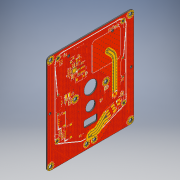
# Autodesk Inventor part: +XPanel_PCB
Saved by Autodesk Inventor 2018 (Build 220112000, 112)
## iProperties
Created: 2018-10-25
Part Number: +XPanel_PCB
Material: Epoxy Resin
Document SubType Name: Modeling
Designer: Bradley
Density: 1.14 g/cm^3
Appearance: Smooth - Dark Gray
Author: Bradley
Autodesk Inventor part; units mm, degrees
ref_plane "YZ Plane" through (0, 0, 0) normal (1, 0, 0) x (0, 1, 0)
ref_plane "XZ Plane" through (0, 0, 0) normal (0, 1, 0) x (-1, 0, 0)
ref_plane "XY Plane" through (0, 0, 0) normal (0, 0, 1) x (1, 0, 0)
sketch "Sketch1" plane through (0, 0, 0) normal (1, 0, 0) x (0, 1, 0)
  line L0 (36.5, -42) -> (-36.5, -42) construction
  line L1 (-36.5, -42) -> (-36.5, 42) construction
  line L2 (-36.5, 42) -> (36.5, 42) construction
  line L3 (36.5, 42) -> (36.5, -42) construction
  line L4 (36.5, -42) -> (-36.5, 42) construction
  line L5 (-36.5, -42) -> (36.5, 42) construction
  line L6 (-14, 0) -> (14, 0) construction
  line L7 (-39.5, -42) -> (-39.5, 42)
  arc A0 (-36.5, 45) -> (-39.5, 42) centre (-36.5, 42) ccw
  line L8 (-36.5, 45) -> (36.5, 45)
  arc A1 (39.5, 42) -> (36.5, 45) centre (36.5, 42) ccw
  line L9 (39.5, 42) -> (39.5, -42)
  arc A2 (36.5, -45) -> (39.5, -42) centre (36.5, -42) ccw
  line L10 (36.5, -45) -> (-36.5, -45)
  arc A3 (-39.5, -42) -> (-36.5, -45) centre (-36.5, -42) ccw
  point P0 (0, 0)
  point P1 (0, 0)
  dimension "d2" = 28
  dimension "d3" = 79
  dimension "d117" = 3
  dimension "d118" = 90
  dimension "d119" = 84
  dimension "d120" = 73
  constraints: 22 end point, 8 point on circle, 6 tangent, 4 centre point, 4 coincident, 4 midpoint, 4 parallel, 2 horizontal, 2 perpendicular, 1 equal radius, 1 vertical
  measures "d2" distance of L6.start L6.end
  measures "d3" distance between parallel lines of L9 L7
  measures "d117" radius of A0
  measures "d118" distance between parallel lines of L10 L8
  measures "d119" distance of L0.end L1.end
  measures "d120" distance of L1.end L2.end
extrude "Extrusion1" add sketch "Sketch1" along normal mid plane 1
sketch "Sketch3" plane through (0.5, 0, 0) normal (1, 0, 0) x (0, 0, -1)
  circle A0 centre (-2.5, 0) radius 6
  circle A1 centre (12.35, 0) radius 4.5
  line L0 (26, -6) -> (22, -6)
  line L1 (21, -5) -> (21, 5)
  line L2 (22, 6) -> (26, 6)
  line L3 (27, 5) -> (27, -5)
  line L4 (27, -6) -> (21, 6) construction
  line L5 (21, -6) -> (27, 6) construction
  arc A2 (21, -5) -> (22, -6) centre (22, -5) ccw
  arc A3 (26, -6) -> (27, -5) centre (26, -5) ccw
  arc A4 (27, 5) -> (26, 6) centre (26, 5) ccw
  arc A5 (22, 6) -> (21, 5) centre (22, 5) ccw
  point P0 (0, 0)
  point P1 (24, 0)
  point P2 (24, 0)
  dimension "d15" = 2.5
  dimension "d16" = 12
  dimension "d17" = 14.85
  dimension "d18" = 9
  dimension "d84" = 24
  dimension "d85" = 12
  dimension "d86" = 6
  dimension "d87" = 1
  constraints: 12 end point, 8 point on circle, 8 point on line, 8 tangent, 6 centre point, 3 equal radius, 3 horizontal alignment, 3 midpoint, 2 parallel, 1 horizontal, 1 perpendicular
  measures "d15" distance of point (0, 0) A0.centre
  measures "d16" diameter of A0
  measures "d17" distance of A1.centre A0.centre
  measures "d18" diameter of A1
  measures "d84" distance of point (0, 0) point (24, 0)
  measures "d85" distance of L5.start L4.end
  measures "d86" distance of L4.start L5.start
  measures "d87" radius of A2
extrude "Extrusion2" cut sketch "Sketch3" against normal through all
sketch "Sketch7" plane through (0.5, 0, 0) normal (1, 0, 0) x (0, 0, -1)
  line L0 (-45, 36.5) -> (-45, -36.5) projected
  line L1 (45, -36.5) -> (45, 36.5) projected
  line L2 (-45, -39.5061) -> (-45, 39.5061) construction
  line L3 (-45, 39.5061) -> (45, 39.5061) construction
  line L4 (45, 39.5061) -> (45, -39.5061) construction
  line L5 (45, -39.5061) -> (-45, -39.5061) construction
  point P0 (0, 0)
  point P1 (-45, 0)
  point P2 (-45, 0)
  constraints: 3 midpoint, 2 collinear, 2 other
decal "Decal2"
sketch "Sketch8" plane through (-0.5, 0, 0) normal (-1, 0, 0) x (0, 0, 1)
  line L0 (45, 39.5061) -> (45, -39.5061) construction
  line L1 (45, -39.5061) -> (-45, -39.5061) construction
  line L2 (-45, -39.5061) -> (-45, 39.5061) construction
  line L3 (-45, 39.5061) -> (45, 39.5061) construction
  line L4 (45, -36.5) -> (45, 36.5) projected
  line L5 (-45, 36.5) -> (-45, -36.5) projected
  point P0 (0, 0)
  point P1 (45, 0)
  constraints: 2 collinear, 2 midpoint, 2 other
decal "Decal3"
sketch "Sketch9" plane through (0.5, 0, 0) normal (1, 0, 0) x (0, 0, -1)
  point P0 (0, 0)
  point P1 (0, -14)
  point P2 (-42, -36.5)
  point P3 (42, -36.5)
  point P4 (42, 36.5)
  point P5 (-42, 36.5)
  point P6 (0, 14)
  constraints: 7 other
hole "Hole7" at (0.5, -14, 0) at (0.5, -36.5, 42) at (0.5, -36.5, -42) at (0.5, 36.5, -42) at (0.5, 36.5, 42) at (0.5, 14, 0) direction (-1, 0, 0) diameter 3.3 end through all
sketch "Sketch10" plane through (0.5, 0, 0) normal (1, 0, 0) x (0, 0, -1)
  point P0 (0, 0)
  point P1 (40.5, 3.5)
  point P2 (40.5, -3.5)
  constraints: 2 other
hole "Hole8" at (0.5, 3.5, -40.5) at (0.5, -3.5, -40.5) direction (-1, 0, 0) diameter 3 end through all
sketch "Sketch11" plane through (0.5, 0, 0) normal (1, 0, 0) x (0, 0, -1)
  line L0 (-37, -20) -> (-37, 20) construction
  line L1 (-34.55, -12.55) -> (-9.45, -12.55) construction
  line L2 (-9.45, -12.55) -> (-9.45, 12.55) construction
  line L3 (-9.45, 12.55) -> (-34.55, 12.55) construction
  line L4 (-34.55, 12.55) -> (-34.55, -12.55) construction
  circle A0 centre (-37, -20) radius 0.75 construction
  circle A1 centre (-37, 20) radius 0.75 construction
  line L5 (36, 6) -> (36, -6) construction
  line L6 (0, 37) -> (0, -37) construction
  point P0 (0, 0)
  point P1 (-37, 0)
  point P2 (-9.45, 0)
  point P3 (36, 0)
  point P4 (0, 0)
  dimension "d225" = 25.1
  dimension "d226" = 9.45
  dimension "d227" = 40
  dimension "d228" = 1.5
  dimension "d229" = 12
  dimension "d230" = 36
  dimension "d231" = 37
  dimension "d233" = 74
  constraints: 14 end point, 4 midpoint, 3 coincident, 3 horizontal alignment, 3 vertical, 2 centre point, 2 parallel, 2 perpendicular, 1 equal radius, 1 horizontal, 1 other
  measures "d225" distance of L3.end L2.end
  measures "d226" distance from line of point (0, 0) L2
  measures "d227" distance of L0.start L0.end
  measures "d228" diameter of A0
  measures "d229" distance of L5.start L5.end
  measures "d230" distance from line of L5 point (0, 0)
  measures "d231" distance from line of point (0, 0) L0
  measures "d233" distance of L6.start L6.end
hole "Hole9" at (0.5, -37, 0) at (0.5, 37, 0) at (0.5, 20, 37) at (0.5, -20, 37) direction (-1, 0, 0) diameter 2.2 end through all
sketch "Sketch12" plane through (0.5, 0, 0) normal (1, 0, 0) x (0, 0, -1)
  point P0 (0, 0)
  point P1 (4, 29.5)
  point P2 (-11, 29.5)
  point P3 (4, -29.5)
  point P4 (-11, -29.5)
  constraints: 5 other
hole "Hole10" at (0.5, 29.5, -4) at (0.5, 29.5, 11) at (0.5, -29.5, -4) at (0.5, -29.5, 11) direction (-1, 0, 0) diameter 1 end through all
sketch "Sketch13" plane through (0.5, 0, 0) normal (1, 0, 0) x (0, 0, -1)
  point P0 (0, 0)
  point P1 (-23.25, 15.75)
  constraints: 2 other
hole "Hole11" at (0.5, 15.75, 23.25) direction (-1, 0, 0) diameter 0.95 end through all
sketch "Sketch14" plane through (0.5, 0, 0) normal (1, 0, 0) x (0, 0, -1)
  point P0 (0, 0)
  point P1 (36, -1)
  point P2 (36, 1)
  constraints: 3 other
hole "Hole12" at (0.5, -1, -36) at (0.5, 1, -36) direction (-1, 0, 0) diameter 0.7 end through all
sketch "Sketch15" plane through (0.5, 0, 0) normal (1, 0, 0) x (0, 0, -1)
  point P0 (0, 0)
  point P1 (1.352, -12.139)
  point P2 (42, -34.2)
  point P3 (40.648, -34.639)
  point P4 (39.813, -35.789)
  point P5 (39.813, -37.211)
  point P6 (40.648, -38.361)
  point P7 (42, -38.8)
  point P8 (43.352, -38.361)
  point P9 (44.187, -37.211)
  point P10 (44.187, -35.789)
  point P11 (43.352, -34.639)
  point P12 (-42, -34.2)
  point P13 (-43.352, -34.639)
  point P14 (-44.187, -35.789)
  point P15 (-44.187, -37.211)
  point P16 (-43.352, -38.361)
  point P17 (-42, -38.8)
  point P18 (-40.648, -38.361)
  point P19 (-39.813, -37.211)
  point P20 (-39.813, -35.789)
  point P21 (-40.648, -34.639)
  point P22 (-42, 38.8)
  point P23 (-43.352, 38.361)
  point P24 (-44.187, 37.211)
  point P25 (-44.187, 35.789)
  point P26 (-43.352, 34.639)
  point P27 (-42, 34.2)
  point P28 (-40.648, 34.639)
  point P29 (-39.813, 37.211)
  point P30 (-40.648, 38.361)
  point P31 (-39.813, 35.789)
  point P32 (42, 38.8)
  point P33 (40.648, 38.361)
  point P34 (39.813, 37.211)
  point P35 (39.813, 35.789)
  point P36 (40.648, 34.639)
  point P37 (42, 34.2)
  point P38 (43.352, 34.639)
  point P39 (44.187, 35.789)
  point P40 (44.187, 37.211)
  point P41 (43.352, 38.361)
  point P42 (0, -11.7)
  point P43 (0, 16.3)
  point P44 (-1.352, 15.861)
  point P45 (-2.187, 14.711)
  point P46 (-2.187, 13.289)
  point P47 (-1.352, 12.139)
  point P48 (0, 11.7)
  point P49 (1.352, 12.139)
  point P50 (2.187, 13.289)
  point P51 (2.187, 14.711)
  point P52 (1.352, 15.861)
  point P53 (-1.352, -12.139)
  point P54 (-2.187, -13.289)
  point P55 (-2.187, -14.711)
  point P56 (-1.352, -15.861)
  point P57 (0, -16.3)
  point P58 (1.352, -15.861)
  point P59 (2.187, -14.711)
  point P60 (40.5, 5.6)
  point P61 (39.015, 4.985)
  point P62 (38.4, 3.5)
  point P63 (39.015, 2.015)
  point P64 (40.5, 1.4)
  point P65 (41.985, 2.015)
  point P66 (42.6, 3.5)
  point P67 (41.985, 4.985)
  point P68 (2.187, -13.289)
  point P69 (40.5, -1.4)
  point P70 (39.015, -2.015)
  point P71 (38.4, -3.5)
  point P72 (39.015, -4.985)
  point P73 (40.5, -5.6)
  point P74 (41.985, -4.985)
  point P75 (42.6, -3.5)
  point P76 (41.985, -2.015)
  constraints: 77 other
hole "Hole13" at (0.5, -12.139, -1.352) at (0.5, -34.2, -42) at (0.5, -34.639, -40.648) at (0.5, -35.789, -39.813) at (0.5, -37.211, -39.813) at (0.5, -38.361, -40.648) at (0.5, -38.8, -42) at (0.5, -38.361, -43.352) at (0.5, -37.211, -44.187) at (0.5, -35.789, -44.187) at (0.5, -34.639, -43.352) at (0.5, -34.2, 42) at (0.5, -34.639, 43.352) at (0.5, -35.789, 44.187) at (0.5, -37.211, 44.187) at (0.5, -38.361, 43.352) at (0.5, -38.8, 42) at (0.5, -38.361, 40.648) at (0.5, -37.211, 39.813) at (0.5, -35.789, 39.813) at (0.5, -34.639, 40.648) at (0.5, 38.8, 42) at (0.5, 38.361, 43.352) at (0.5, 37.211, 44.187) at (0.5, 35.789, 44.187) at (0.5, 34.639, 43.352) at (0.5, 34.2, 42) at (0.5, 34.639, 40.648) at (0.5, 37.211, 39.813) at (0.5, 38.361, 40.648) at (0.5, 35.789, 39.813) at (0.5, 38.8, -42) at (0.5, 38.361, -40.648) at (0.5, 37.211, -39.813) at (0.5, 35.789, -39.813) at (0.5, 34.639, -40.648) at (0.5, 34.2, -42) at (0.5, 34.639, -43.352) at (0.5, 35.789, -44.187) at (0.5, 37.211, -44.187) at (0.5, 38.361, -43.352) at (0.5, -11.7, 0) at (0.5, 16.3, 0) at (0.5, 15.861, 1.352) at (0.5, 14.711, 2.187) at (0.5, 13.289, 2.187) at (0.5, 12.139, 1.352) at (0.5, 11.7, 0) at (0.5, 12.139, -1.352) at (0.5, 13.289, -2.187) direction (-1, 0, 0) diameter 0.45 end through all and at (0.5, 14.711, -2.187) (0.5, 15.861, -1.352) (0.5, -12.139, 1.352) (0.5, -13.289, 2.187) (0.5, -14.711, 2.187) (0.5, -15.861, 1.352) (0.5, -16.3, 0) (0.5, -15.861, -1.352) (0.5, -14.711, -2.187) (0.5, 5.6, -40.5) (0.5, 4.985, -39.015) (0.5, 3.5, -38.4) (0.5, 2.015, -39.015) (0.5, 1.4, -40.5) (0.5, 2.015, -41.985) (0.5, 3.5, -42.6) (0.5, 4.985, -41.985) (0.5, -13.289, -2.187) (0.5, -1.4, -40.5) (0.5, -2.015, -39.015) (0.5, -3.5, -38.4) (0.5, -4.985, -39.015) (0.5, -5.6, -40.5) (0.5, -4.985, -41.985) (0.5, -3.5, -42.6) (0.5, -2.015, -41.985)
sketch "Sketch16" plane through (0.5, 0, 0) normal (1, 0, 0) x (0, 0, -1)
  point P0 (0, 0)
  point P1 (1.6, 23.6)
  point P2 (0.4, 23.6)
  point P3 (-0.8, 23.6)
  point P4 (-2, 23.6)
  point P5 (-3.2, 23.6)
  point P6 (-4.4, 23.6)
  point P7 (-5.6, 23.6)
  point P8 (-6.8, 23.6)
  point P9 (-8, 23.6)
  point P10 (-9.2, 23.6)
  point P11 (-10.4, 23.6)
  point P12 (11.3, 20.4)
  point P13 (10.1, 20.4)
  point P14 (8.9, 20.4)
  point P15 (7.7, 20.4)
  point P16 (6.5, 20.4)
  point P17 (5.3, 20.4)
  point P18 (4.1, 20.4)
  point P19 (2.9, 20.4)
  point P20 (1.7, 20.4)
  point P21 (0.5, 20.4)
  point P22 (-0.7, 20.4)
  point P23 (-1.9, 20.4)
  point P24 (-3.1, 20.4)
  point P25 (-4.3, 20.4)
  point P26 (-5.5, 20.4)
  point P27 (-6.7, 20.4)
  point P28 (-7.9, 20.4)
  point P29 (-9.1, 20.4)
  point P30 (-10.3, 20.4)
  point P31 (-11.5, 20.4)
  point P32 (-12.7, 20.4)
  point P33 (-11.6, 23.6)
  point P34 (-12.8, 23.6)
  point P35 (-13.9, 20.3)
  point P36 (-15.1, 20.1)
  point P37 (-16.2, 19.7)
  point P38 (-17.3, 19.1)
  point P39 (-18.3, 18.4)
  point P40 (-19.1, 17.6)
  point P41 (-19.9, 16.8)
  point P42 (-20.7, 16)
  point P43 (-21.5, 15.2)
  point P44 (-22.2, 14.2)
  point P45 (-23.4, 13.9)
  point P46 (-24.5, 14.4)
  point P47 (-25.1, 15.4)
  point P48 (-24.9, 16.6)
  point P49 (-24, 17.4)
  point P50 (-23.1, 18.2)
  point P51 (-22.3, 19)
  point P52 (-21.5, 19.8)
  point P53 (-20.7, 20.6)
  point P54 (-19.8, 21.3)
  point P55 (-18.8, 22)
  point P56 (-17.8, 22.5)
  point P57 (-16.6, 23.1)
  point P58 (-15.5, 23.4)
  point P59 (-14.2, 23.6)
  point P60 (12.5, 20.5)
  point P61 (12.5, 23.5)
  point P62 (10, 18)
  point P63 (14, 18)
  point P64 (16, 20)
  point P65 (16, 24)
  point P66 (14, 26)
  point P67 (10, 26)
  point P68 (6, 18)
  point P69 (2, 18)
  point P70 (-2, 18)
  point P71 (6, 26)
  point P72 (2, 26)
  point P73 (-2, 26)
  point P74 (-6, 26)
  point P75 (-10, 26)
  point P76 (-14, 26)
  point P77 (-18, 26)
  point P78 (-22, 26)
  point P79 (-26, 26)
  point P80 (-30, 26)
  point P81 (-34, 26)
  point P82 (-24, 24)
  point P83 (-28, 24)
  point P84 (-32, 24)
  point P85 (-36, 24)
  point P86 (-22, 22)
  point P87 (-26, 22)
  point P88 (-30, 22)
  point P89 (-34, 22)
  point P90 (-24, 20)
  point P91 (-28, 20)
  point P92 (-32, 20)
  point P93 (-36, 20)
  point P94 (-36, 16)
  point P95 (-36, 12)
  point P96 (-36, 8)
  point P97 (-36, 4)
  point P98 (-34, 18)
  point P99 (20, 16)
  point P100 (-34, 10)
  point P101 (-34, 6)
  point P102 (-34, 2)
  point P103 (-32, 16)
  point P104 (-32, 12)
  point P105 (-32, 8)
  point P106 (-32, 4)
  point P107 (-30, 18)
  point P108 (-30, 14)
  point P109 (-30, 10)
  point P110 (-30, 6)
  point P111 (-30, 2)
  point P112 (-28, 16)
  point P113 (-28, 12)
  point P114 (-28, 8)
  point P115 (-28, 4)
  point P116 (-26, 18)
  point P117 (-26, 14)
  point P118 (-26, 10)
  point P119 (-26, 6)
  point P120 (-26, 2)
  point P121 (-24, 12)
  point P122 (-24, 8)
  point P123 (-24, 4)
  point P124 (-22, 10)
  point P125 (-22, 6)
  point P126 (-22, 2)
  point P127 (-20, 12)
  point P128 (-20, 8)
  point P129 (-20, 4)
  point P130 (-18, 14)
  point P131 (-18, 10)
  point P132 (-18, 6)
  point P133 (-18, 2)
  point P134 (-16, 16)
  point P135 (-16, 12)
  point P136 (-16, 8)
  point P137 (-16, 4)
  point P138 (-14, 14)
  point P139 (-14, 10)
  point P140 (-14, 6)
  point P141 (-14, 2)
  point P142 (-14, 18)
  point P143 (-12, 16)
  point P144 (-10, 18)
  point P145 (-12, 12)
  point P146 (-10, 14)
  point P147 (-8, 16)
  point P148 (-12, 8)
  point P149 (-10, 10)
  point P150 (-8, 12)
  point P151 (-6, 14)
  point P152 (-4, 16)
  point P153 (-6, 18)
  point P154 (-20, 24)
  point P155 (19.2, 29.2)
  point P156 (10.9, -11.3)
  point P157 (-37.8, -27.3)
  point P158 (3.6, -27.3)
  point P159 (33.2, 33.6)
  point P160 (34.2, 36.1)
  point P161 (11, -26.9)
  point P162 (3.2, -22.9)
  point P163 (-17.2, -10.5)
  point P164 (-17.2, -7.3)
  point P165 (11, -21.9)
  point P166 (-2.1, -24.2)
  point P167 (25, 31.989)
  point P168 (23.869, 31.521)
  point P169 (23.4, 30.389)
  point P170 (23.869, 29.258)
  point P171 (25, 28.789)
  point P172 (26.131, 29.258)
  point P173 (26.6, 30.389)
  point P174 (26.131, 31.521)
  point P175 (-27.6, -11.9)
  point P176 (-28, -13.7)
  point P177 (8.3, 29.9)
  point P178 (-3.9, -16.4)
  point P179 (12.7, -20.7)
  point P180 (-0.7, -21)
  point P181 (9.8, 11.1)
  point P182 (-14.6, -14.2)
  point P183 (-27.1, -9.405)
  point P184 (-24.77, -11.5)
  point P185 (-25.164, -17.236)
  point P186 (-25.18, -12.4)
  point P187 (-40, -27.996)
  point P188 (-41.131, -28.465)
  point P189 (-41.6, -29.596)
  point P190 (-41.131, -30.727)
  point P191 (-40, -31.196)
  point P192 (-38.869, -30.727)
  point P193 (-38.4, -29.596)
  point P194 (-38.869, -28.465)
  point P195 (-29.7, -17.5)
  point P196 (25, -28.789)
  point P197 (23.869, -29.258)
  point P198 (23.4, -30.389)
  point P199 (23.869, -31.521)
  constraints: 292 other
hole "Hole14" at (0.5, 23.6, -1.6) at (0.5, 23.6, -0.4) at (0.5, 23.6, 0.8) at (0.5, 23.6, 2) at (0.5, 23.6, 3.2) at (0.5, 23.6, 4.4) at (0.5, 23.6, 5.6) at (0.5, 23.6, 6.8) at (0.5, 23.6, 8) at (0.5, 23.6, 9.2) at (0.5, 23.6, 10.4) at (0.5, 20.4, -11.3) at (0.5, 20.4, -10.1) at (0.5, 20.4, -8.9) at (0.5, 20.4, -7.7) at (0.5, 20.4, -6.5) at (0.5, 20.4, -5.3) at (0.5, 20.4, -4.1) at (0.5, 20.4, -2.9) at (0.5, 20.4, -1.7) at (0.5, 20.4, -0.5) at (0.5, 20.4, 0.7) at (0.5, 20.4, 1.9) at (0.5, 20.4, 3.1) at (0.5, 20.4, 4.3) at (0.5, 20.4, 5.5) at (0.5, 20.4, 6.7) at (0.5, 20.4, 7.9) at (0.5, 20.4, 9.1) at (0.5, 20.4, 10.3) at (0.5, 20.4, 11.5) at (0.5, 20.4, 12.7) at (0.5, 23.6, 11.6) at (0.5, 23.6, 12.8) at (0.5, 20.3, 13.9) at (0.5, 20.1, 15.1) at (0.5, 19.7, 16.2) at (0.5, 19.1, 17.3) at (0.5, 18.4, 18.3) at (0.5, 17.6, 19.1) at (0.5, 16.8, 19.9) at (0.5, 16, 20.7) at (0.5, 15.2, 21.5) at (0.5, 14.2, 22.2) at (0.5, 13.9, 23.4) at (0.5, 14.4, 24.5) at (0.5, 15.4, 25.1) at (0.5, 16.6, 24.9) at (0.5, 17.4, 24) at (0.5, 18.2, 23.1) direction (-1, 0, 0) diameter 0.35 end through all and at (0.5, 19, 22.3) (0.5, 19.8, 21.5) (0.5, 20.6, 20.7) (0.5, 21.3, 19.8) (0.5, 22, 18.8) (0.5, 22.5, 17.8) (0.5, 23.1, 16.6) (0.5, 23.4, 15.5) (0.5, 23.6, 14.2) (0.5, 20.5, -12.5) (0.5, 23.5, -12.5) (0.5, 18, -10) (0.5, 18, -14) (0.5, 20, -16) (0.5, 24, -16) (0.5, 26, -14) (0.5, 26, -10) (0.5, 18, -6) (0.5, 18, -2) (0.5, 18, 2) (0.5, 26, -6) (0.5, 26, -2) (0.5, 26, 2) (0.5, 26, 6) (0.5, 26, 10) (0.5, 26, 14) (0.5, 26, 18) (0.5, 26, 22) (0.5, 26, 26) (0.5, 26, 30) (0.5, 26, 34) (0.5, 24, 24) (0.5, 24, 28) (0.5, 24, 32) (0.5, 24, 36) (0.5, 22, 22) (0.5, 22, 26) (0.5, 22, 30) (0.5, 22, 34) (0.5, 20, 24) (0.5, 20, 28) (0.5, 20, 32) (0.5, 20, 36) (0.5, 16, 36) (0.5, 12, 36) (0.5, 8, 36) (0.5, 4, 36) (0.5, 18, 34) (0.5, 16, -20) (0.5, 10, 34) (0.5, 6, 34) (0.5, 2, 34) (0.5, 16, 32) (0.5, 12, 32) (0.5, 8, 32) (0.5, 4, 32) (0.5, 18, 30) (0.5, 14, 30) (0.5, 10, 30) (0.5, 6, 30) (0.5, 2, 30) (0.5, 16, 28) (0.5, 12, 28) (0.5, 8, 28) (0.5, 4, 28) (0.5, 18, 26) (0.5, 14, 26) (0.5, 10, 26) (0.5, 6, 26) (0.5, 2, 26) (0.5, 12, 24) (0.5, 8, 24) (0.5, 4, 24) (0.5, 10, 22) (0.5, 6, 22) (0.5, 2, 22) (0.5, 12, 20) (0.5, 8, 20) (0.5, 4, 20) (0.5, 14, 18) (0.5, 10, 18) (0.5, 6, 18) (0.5, 2, 18) (0.5, 16, 16) (0.5, 12, 16) (0.5, 8, 16) (0.5, 4, 16) (0.5, 14, 14) (0.5, 10, 14) (0.5, 6, 14) (0.5, 2, 14) (0.5, 18, 14) (0.5, 16, 12) (0.5, 18, 10) (0.5, 12, 12) (0.5, 14, 10) (0.5, 16, 8) (0.5, 8, 12) (0.5, 10, 10) (0.5, 12, 8) (0.5, 14, 6) (0.5, 16, 4) (0.5, 18, 6) (0.5, 24, 20) (0.5, 29.2, -19.2) (0.5, -11.3, -10.9) (0.5, -27.3, 37.8) (0.5, -27.3, -3.6) (0.5, 33.6, -33.2) (0.5, 36.1, -34.2) (0.5, -26.9, -11) (0.5, -22.9, -3.2) (0.5, -10.5, 17.2) (0.5, -7.3, 17.2) (0.5, -21.9, -11) (0.5, -24.2, 2.1) (0.5, 31.989, -25) (0.5, 31.521, -23.869) (0.5, 30.389, -23.4) (0.5, 29.258, -23.869) (0.5, 28.789, -25) (0.5, 29.258, -26.131) (0.5, 30.389, -26.6) (0.5, 31.521, -26.131) (0.5, -11.9, 27.6) (0.5, -13.7, 28) (0.5, 29.9, -8.3) (0.5, -16.4, 3.9) (0.5, -20.7, -12.7) (0.5, -21, 0.7) (0.5, 11.1, -9.8) (0.5, -14.2, 14.6) (0.5, -9.405, 27.1) (0.5, -11.5, 24.77) (0.5, -17.236, 25.164) (0.5, -12.4, 25.18) (0.5, -27.996, 40) (0.5, -28.465, 41.131) (0.5, -29.596, 41.6) (0.5, -30.727, 41.131) (0.5, -31.196, 40) (0.5, -30.727, 38.869) (0.5, -29.596, 38.4) (0.5, -28.465, 38.869) (0.5, -17.5, 29.7) (0.5, -28.789, -25) (0.5, -29.258, -23.869) (0.5, -30.389, -23.4) (0.5, -31.521, -23.869) (0.5, -31.989, -25) (0.5, -31.521, -26.131) (0.5, -30.389, -26.6) (0.5, -29.258, -26.131) (0.5, -16.5, 25.765) (0.5, 31.196, 40) (0.5, 30.727, 41.131) (0.5, 29.596, 41.6) (0.5, 28.465, 41.131) (0.5, 27.996, 40) (0.5, 28.465, 38.869) (0.5, 29.596, 38.4) (0.5, 30.727, 38.869) (0.5, -15.7, 8.6) (0.5, -19.2, 32.5) (0.5, -17.8, 33.9) (0.5, -16.6, 16.7) (0.5, -23, -18.1) (0.5, -20.4, 19.9) (0.5, -15.8, 7.1) (0.5, -21.1, -25.3) (0.5, -17.665, 22.515) (0.5, -17.214, 21.785) (0.5, -18.6, -23.7) (0.5, -34.1, -29.4) (0.5, -15.7, 31.7) (0.5, -13.9, 29.015) (0.5, -12.9, 18.4) (0.5, -23.8, 8.7) (0.5, -18.384, 13.289) (0.5, -14.3, 16.2) (0.5, 16.5, -8.8) (0.5, -9.6, 16.4) (0.5, -8.8, -1.5) (0.5, -9.9, 1) (0.5, 8.9, -5) (0.5, -9.042, 22.515) (0.5, -19.4, 38.3) (0.5, -7.814, 22.986) (0.5, -3.9, 36.4) (0.5, -6.514, 23.286) (0.5, -9.4, 25.5) (0.5, -10.012, 24.185) (0.5, 14, 34) (0.5, 12, -24) (0.5, 14, -22) (0.5, 20, -20) (0.5, 10, -26) (0.5, 8, -28) (0.5, 6, -30) (0.5, 4, -32) (0.5, 0, -32) (0.5, 2, -30) (0.5, 4, -28) (0.5, 0, -28) (0.5, -2, -30) (0.5, -4, -32) (0.5, -6, -34) (0.5, -6, -38) (0.5, -4, -36) (0.5, -2, -34) (0.5, 24, -20) (0.5, 28, -20) (0.5, 27.8, -23.9) (0.5, 26, -26) (0.5, 24, -28) (0.5, 22, -30) (0.5, 24, -24) (0.5, 20, -28) (0.5, 20, -32) (0.5, 18, -34) (0.5, 16, -36) (0.5, 14, -38) (0.5, 12, -40) (0.5, 10, -42) (0.5, 8, -40) (0.5, 10, -38) (0.5, 12, -36) (0.5, 14, -34) (0.5, 16, -32) (0.5, 12, -32) (0.5, 10, -34) (0.5, 8, -36) (0.5, 6, -38) (0.5, 23.6, -11.2) (0.5, 23.6, -10) (0.5, 23.6, -8.8) (0.5, 23.6, -7.6) (0.5, 23.6, -6.4) (0.5, 23.6, -5.2) (0.5, 23.6, -4) (0.5, 23.6, -2.8)
body "Solid1"
